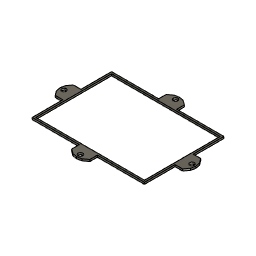
blimp_PCB (Autodesk Fusion 360 archive; units mm, degrees)
design "drzak_kamera"
Autodesk Fusion 360 part; units mm, degrees
(part 1 of 2)
sketch "Sketch1" plane through (0, 0, 0) normal (0, 0, 1) x (1, 0, 0)
  line L0 (29.9, -20.85) -> (-29.9, -20.85)
  line L1 (-29.9, -20.85) -> (-29.9, 20.85)
  line L2 (-29.9, 20.85) -> (29.9, 20.85)
  line L3 (29.9, 20.85) -> (29.9, -20.85)
  line L4 (29.9, -20.85) -> (-29.9, 20.85) construction
  line L5 (-29.9, -20.85) -> (29.9, 20.85) construction
  line L6 (30.9, -21.85) -> (-30.9, -21.85)
  line L7 (-30.9, -21.85) -> (-30.9, 21.85)
  line L8 (-30.9, 21.85) -> (30.9, 21.85)
  line L9 (30.9, 21.85) -> (30.9, -21.85)
  line L10 (30.9, -21.85) -> (-30.9, 21.85) construction
  line L11 (-30.9, -21.85) -> (30.9, 21.85) construction
  dimension "d5" = 41.7
  dimension "d6" = 59.8
  dimension "d8" = 1
  dimension "d9" = 1
  constraint horizontal L0
  constraint perpendicular L0 L1
  constraint parallel L0 L2
  constraint parallel L1 L3
  constraint coincident L4 origin
  constraint coincident L5 origin
  constraint horizontal L6
  constraint perpendicular L6 L7
  constraint parallel L6 L8
  constraint parallel L7 L9
  constraint coincident L10 origin
  constraint coincident L11 origin
  measures "d5" distance of L0 L2
  measures "d6" distance of L1 L3
  measures "d8" distance of L3 L9
  measures "d9" distance of L2 L8
extrude "Extrude1" add sketch "Sketch1" along normal blind 20 makes body 1
extrude "Extrude2" add sketch "Sketch1" against normal blind 1 contours L0 L1 L2 L3 | L6 L7 L8 L9 bodies 1
sketch "Sketch2" plane through (0, 0, -1) normal (0, 0, -1) x (1, 0, 0)
  line L0 (-30.9, -21.85) -> (30.9, -21.85)
  line L1 (30.9, -21.85) -> (30.9, 21.85)
  line L2 (30.9, 21.85) -> (-30.9, 21.85)
  line L3 (-30.9, 21.85) -> (-30.9, -21.85)
  line L4 (29.9, -20.85) -> (29.9, 20.85)
  line L5 (29.9, 20.85) -> (-29.9, 20.85)
  line L6 (-29.9, -20.85) -> (29.9, -20.85)
  line L7 (-29.9, 20.85) -> (-29.9, -20.85)
  circle A0 centre (-14.1, -6.05) radius 10.8
  line L8 (-14.1, -6.05) -> (-14.1, -20.1) construction
  line L9 (-14.1, -6.05) -> (-11.3071, -6.05) construction
  line L10 (-14.1, -6.05) -> (-26.7, -6.05) construction
  point P0 (-14.1, -16.85)
  point P1 (-24.9, -6.05)
  dimension "d16" = 4
  dimension "d18" = 21.6
  dimension "d22" = 5
  constraint coincident A0.centre L8.start
  constraint perpendicular L0 L8
  constraint coincident A0 P0
  constraint coincident L8 P0
  constraint perpendicular L8 L9
  constraint perpendicular L8 L10
  constraint coincident A0 P1
  constraint coincident L10 P1
  measures "d16" distance of L6 P0
  measures "d18" diameter of A0
  measures "d22" distance of L7 P1
extrude "Extrude3" cut sketch "Sketch2" against normal blind 10 contours A0 bodies 1
sketch "Sketch4" plane through (0, 0, 20) normal (0, 0, 1) x (-1, 0, 0)
  line L0 (29.9, -20.85) -> (-29.9, -20.85)
  line L1 (-29.9, -20.85) -> (-29.9, 20.85)
  line L2 (-29.9, 20.85) -> (29.9, 20.85)
  line L3 (29.9, 20.85) -> (29.9, -20.85)
  line L4 (-30.9, -21.85) -> (30.9, -21.85)
  line L5 (30.9, -21.85) -> (30.9, 21.85)
  line L6 (30.9, 21.85) -> (-30.9, 21.85)
  line L7 (-30.9, 21.85) -> (-30.9, -21.85)
  circle A0 centre (0, 21.85) radius 6.5 construction
  line L8 (5, 21.85) -> (5, 29.4381)
  line L9 (0, 21.85) -> (0, 31.6147) construction
  line L10 (-5, 21.85) -> (-5, 29.4381)
  line L11 (0, 0) -> (38, 0) construction
  circle A1 centre (30.9, 0) radius 6.5
  line L12 (30.9, 5) -> (35.0533, 5)
  line L13 (30.9, -5) -> (35.0533, -5)
  circle A2 centre (0, 26.1833) radius 1.25
  line L14 (-30.9, 21.85) -> (30.9, 21.85)
  circle A3 centre (35.2333, 0) radius 1.25
  line L15 (30.9, 21.85) -> (30.9, -21.85)
  line L16 (0, 28.35) -> (2.5, 27.85)
  line L17 (2.5, 27.85) -> (5, 26.0033)
  line L18 (-2.5, 27.85) -> (-5, 26.0033)
  line L19 (0, 28.35) -> (-2.5, 27.85)
  line L20 (37.4, 0) -> (36.9, 2.5)
  line L21 (36.9, 2.5) -> (35.0533, 5)
  line L22 (37.4, 0) -> (36.9, -2.5)
  line L23 (36.9, -2.5) -> (35.0533, -5)
  line L24 (-5, -21.85) -> (-5, -29.4381)
  line L25 (5, -21.85) -> (5, -29.4381)
  line L26 (2.5, -27.85) -> (5, -26.0033)
  line L27 (0, -28.35) -> (2.5, -27.85)
  line L28 (0, -28.35) -> (-2.5, -27.85)
  line L29 (-2.5, -27.85) -> (-5, -26.0033)
  circle A4 centre (0, -26.1833) radius 1.25
  line L30 (0, 0) -> (0, -18) construction
  line L31 (-36.9, -2.5) -> (-35.0533, -5)
  line L32 (-37.4, 0) -> (-36.9, -2.5)
  line L33 (-37.4, 0) -> (-36.9, 2.5)
  line L34 (-36.9, 2.5) -> (-35.0533, 5)
  line L35 (-30.9, 5) -> (-35.0533, 5)
  line L36 (-30.9, -5) -> (-35.0533, -5)
  circle A5 centre (-35.2333, 0) radius 1.25
  dimension "d64" = 13
  dimension "d65" = 5
  dimension "d66" = 5
  dimension "d67" = 13
  dimension "d108" = 4.3333
  dimension "d110" = 4.3333
  dimension "d111" = 2.5
  dimension "d136" = 2.5
  dimension "d137" = 2.5
  dimension "d138" = 2.5
  constraint midpoint L6 A0.centre
  constraint coincident L6 L8.start
  constraint perpendicular L6 L8
  constraint coincident A0.centre L9.start
  constraint perpendicular L6 L9
  constraint symmetric L8.start L9 L10.start
  constraint symmetric L8.end L9 L10.end
  constraint coincident L11.start L30.start
  constraint perpendicular L5 L11
  constraint midpoint L5 A1.centre
  constraint coincident L5 L12.start
  constraint perpendicular L5 L12
  constraint symmetric L11 L12.start L13.start
  constraint symmetric L11 L12.end L13.end
  constraint coincident L9 A2.centre
  constraint coincident L11 A3.centre
  constraint coincident A0 L16.start
  constraint coincident L9 L16.start
  constraint coincident A0 L16.end
  constraint coincident L8 L17.end
  constraint coincident A0 L17.end
  constraint symmetric L9 L16.start L19.start
  constraint symmetric L9 L16.end L18.start
  constraint symmetric L9 L17.end L18.end
  constraint coincident A1 L20.start
  constraint coincident L11 L20.start
  constraint coincident A1 L20.end
  constraint coincident A1 L12.end
  constraint symmetric L11 L20.start L22.start
  constraint symmetric L11 L20.end L22.end
  constraint symmetric L8.start L11 L25.start
  constraint symmetric L8.end L11 L25.end
  constraint symmetric L10.start L11 L24.start
  constraint symmetric L10.end L11 L24.end
  constraint symmetric L11 A2 A4
  constraint symmetric L11 L16.start L27.start
  constraint symmetric L11 L16.end L26.start
  constraint symmetric L11 L17.end L26.end
  constraint symmetric L11 L18.start L28.end
  constraint symmetric L11 L18.end L29.end
  constraint perpendicular L11 L30
  constraint symmetric L12.start L30 L35.start
  constraint symmetric L12.end L30 L34.end
  constraint symmetric L13.start L30 L36.start
  constraint symmetric L13.end L30 L31.end
  constraint symmetric A3 L30 A5
  constraint symmetric L20.start L30 L32.start
  constraint symmetric L20.end L30 L33.end
  constraint symmetric L22.end L30 L31.start
  measures "d64" diameter of A0
  measures "d65" distance of L8 L9
  measures "d66" distance of L11 L12
  measures "d67" diameter of A1
  measures "d108" distance of A2.centre L14
  measures "d110" distance of A3.centre L15
  measures "d111" diameter of A3
  measures "d136" diameter of A2
  measures "d137" horizontal distance of L16.start L16.end
  measures "d138" vertical distance of L20.start L20.end
extrude "Extrude5" add sketch "Sketch4" against normal blind 2 contours L5 L12 L13 L15 L20 L21 L22 L23 | L4 L24 L25 L26 L27 L28 L29 | L6 L8 L10 L14 L16 L17 L18 L19 | L7 L31 L32 L33 L34 L35 L36 bodies 1
sketch "Sketch9" plane through (0, 0, 0) normal (0, 0, 1) x (1, 0, 0)
  circle A0 centre (-14.1, 6.05) radius 10.8
sketch "Sketch11" plane through (0, 0, 0) normal (0, 0, 1) x (-1, 0, 0)
  circle A0 centre (14.1, -6.05) radius 10.8
  line L0 (29.9, -20.85) -> (29.9, 20.85)
  line L1 (29.9, 20.85) -> (-29.9, 20.85)
  line L2 (-29.9, 20.85) -> (-29.9, -20.85)
  line L3 (-29.9, -20.85) -> (29.9, -20.85)
  line L4 (-17.7, -20.85) -> (-17.7, 20.85) construction
  line L5 (-38, -7.65) -> (9, -7.65) construction
  circle A1 centre (-17.7, -7.65) radius 5.5
  dimension "d139" = 12.2
  dimension "d140" = 13.2
  dimension "d141" = 11
  constraint coincident L3 L4.start
  constraint coincident L1 L4.end
  constraint perpendicular L1 L4
  constraint perpendicular L4 L5
  constraint coincident L5 A1.centre
  constraint coincident L4 A1.centre
  measures "d139" distance of L2 L4
  measures "d140" distance of L3 L5
  measures "d141" diameter of A1
extrude "Extrude9" cut sketch "Sketch11" against normal blind 1 contours A1 bodies 1
sketch "Sketch12" plane through (0, 20.85, 0) normal (0, -1, 0) x (1, 0, 0)
  line L0 (-29.9, 0) -> (29.9, 0)
  line L1 (29.9, 0) -> (29.9, 20)
  line L2 (29.9, 20) -> (-29.9, 20)
  line L3 (-29.9, 20) -> (-29.9, 0)
  line L4 (18.2, 24) -> (18.2, -6) construction
  line L5 (6, 12.3) -> (38.4279, 12.3) construction
  circle A0 centre (18.2, 12.3) radius 5.5
  dimension "d144" = 11.7
  dimension "d147" = 12.3
  dimension "d148" = 11
  constraint perpendicular L0 L4
  constraint perpendicular L1 L5
  constraint coincident L5 A0.centre
  constraint coincident L4 A0.centre
  measures "d144" distance of L1 L4
  measures "d147" distance of L0 L5
  measures "d148" diameter of A0
extrude "Extrude10" cut sketch "Sketch12" against normal blind 1 contours A0 bodies 1
sketch "Sketch13" plane through (0, 0, 0) normal (0, 0, 1) x (-1, 0, 0)
  circle A0 centre (-17.7, -7.65) radius 5.5
  circle A1 centre (14.1, -6.05) radius 10.8
  line L0 (29.9, -20.85) -> (29.9, 20.85)
  line L1 (29.9, 20.85) -> (-29.9, 20.85)
  line L2 (-29.9, 20.85) -> (-29.9, -20.85)
  line L3 (-29.9, -20.85) -> (29.9, -20.85)
  circle A2 centre (-17.7, -7.65) radius 5.5
  circle A3 centre (14.1, -6.05) radius 10.8
  circle A4 centre (14.1, -6.05) radius 11.8
  circle A5 centre (-17.7, -7.65) radius 6.5
  line L4 (28.4, -20.85) -> (28.4, 20.85)
  line L5 (25.06, -20.85) -> (25.06, 20.85)
  line L6 (24.31, -20.85) -> (24.31, 20.85) construction
  line L7 (20.22, -20.85) -> (20.22, 20.85)
  line L8 (23.56, -20.85) -> (23.56, 20.85)
  line L9 (19.47, -20.85) -> (19.47, 20.85) construction
  line L10 (18.72, -20.85) -> (18.72, 20.85)
  line L11 (15.38, -20.85) -> (15.38, 20.85)
  line L12 (13.88, -20.85) -> (13.88, 20.85)
  line L13 (10.54, -20.85) -> (10.54, 20.85)
  line L14 (9.79, -20.85) -> (9.79, 20.85) construction
  line L15 (9.04, -20.85) -> (9.04, 20.85)
  line L16 (5.7, -20.85) -> (5.7, 20.85)
  line L17 (4.2, -20.85) -> (4.2, 20.85)
  line L18 (0.86, -20.85) -> (0.86, 20.85)
  line L19 (-0.64, -20.85) -> (-0.64, 20.85)
  line L20 (-3.98, -20.85) -> (-3.98, 20.85)
  line L21 (-5.48, -20.85) -> (-5.48, 20.85)
  line L22 (-8.82, -20.85) -> (-8.82, 20.85)
  line L23 (-9.57, -20.85) -> (-9.57, 20.85) construction
  line L24 (-10.32, -20.85) -> (-10.32, 20.85)
  line L25 (-13.66, -20.85) -> (-13.66, 20.85)
  line L26 (-15.16, -20.85) -> (-15.16, 20.85)
  line L27 (-18.5, -20.85) -> (-18.5, 20.85)
  line L28 (-20, -20.85) -> (-20, 20.85)
  line L29 (-23.34, -20.85) -> (-23.34, 20.85)
  line L30 (-24.84, -20.85) -> (-24.84, 20.85)
  line L31 (-28.18, -20.85) -> (-28.18, 20.85)
  line L32 (29.9, -19.35) -> (-29.9, -19.35)
  line L33 (29.9, -15.825) -> (-29.9, -15.825)
  line L34 (29.9, -15.075) -> (-29.9, -15.075) construction
  line L35 (29.9, -10.8) -> (-29.9, -10.8)
  line L36 (29.9, -14.325) -> (-29.9, -14.325)
  line L37 (29.9, -10.05) -> (-29.9, -10.05) construction
  line L38 (29.9, -9.3) -> (-29.9, -9.3)
  line L39 (29.9, -5.775) -> (-29.9, -5.775)
  line L40 (29.9, -5.025) -> (-29.9, -5.025) construction
  line L41 (29.9, -4.275) -> (-29.9, -4.275)
  line L42 (29.9, -0.75) -> (-29.9, -0.75)
  line L43 (29.9, 0.75) -> (-29.9, 0.75)
  line L44 (29.9, 4.275) -> (-29.9, 4.275)
  line L45 (29.9, 5.025) -> (-29.9, 5.025) construction
  line L46 (29.9, 5.775) -> (-29.9, 5.775)
  line L47 (29.9, 9.3) -> (-29.9, 9.3)
  line L48 (29.9, 10.8) -> (-29.9, 10.8)
  line L49 (29.9, 14.325) -> (-29.9, 14.325)
  line L50 (29.9, 15.825) -> (-29.9, 15.825)
  line L51 (29.9, 19.35) -> (-29.9, 19.35)
  line L52 (29.9, 20.1) -> (-29.9, 20.1) construction
  dimension "d151" = 1
  dimension "d152" = 1
  dimension "d155" = 1.5
  dimension "d156" = 3.34
  dimension "d157" = 0.75
  dimension "d158" = 0.75
  dimension "d159" = 0.75
  dimension "d160" = 0.75
  dimension "d161" = 1.5
  dimension "d162" = 1.5
  dimension "d163" = 3.34
  dimension "d164" = 3.34
  dimension "d165" = 5.06
  dimension "d166" = 3.34
  dimension "d167" = 1.5
  dimension "d168" = 3.525
  dimension "d169" = 0.75
  dimension "d170" = 0.75
  constraint coincident L3 L4.start
  constraint coincident L1 L4.end
  constraint perpendicular L1 L4
  constraint coincident L3 L5.start
  constraint coincident L1 L5.end
  constraint perpendicular L1 L5
  constraint coincident L3 L6.start
  constraint coincident L1 L6.end
  constraint perpendicular L1 L6
  constraint symmetric L4.start L6 L7.start
  constraint symmetric L4.end L6 L7.end
  constraint symmetric L5.start L6 L8.start
  constraint symmetric L5.end L6 L8.end
  constraint coincident L3 L9.start
  constraint coincident L1 L9.end
  constraint perpendicular L1 L9
  constraint symmetric L4.start L9 L13.start
  constraint symmetric L4.end L9 L13.end
  constraint symmetric L5.start L9 L12.start
  constraint symmetric L5.end L9 L12.end
  constraint symmetric L7.start L9 L10.start
  constraint symmetric L7.end L9 L10.end
  constraint symmetric L8.start L9 L11.start
  constraint symmetric L8.end L9 L11.end
  constraint coincident L3 L14.start
  constraint coincident L1 L14.end
  constraint perpendicular L1 L14
  constraint symmetric L4.start L14 L22.start
  constraint symmetric L4.end L14 L22.end
  constraint symmetric L5.start L14 L21.start
  constraint symmetric L5.end L14 L21.end
  constraint symmetric L7.start L14 L19.start
  constraint symmetric L7.end L14 L19.end
  constraint symmetric L8.start L14 L20.start
  constraint symmetric L8.end L14 L20.end
  constraint symmetric L10.start L14 L18.start
  constraint symmetric L10.end L14 L18.end
  constraint symmetric L11.start L14 L17.start
  constraint symmetric L11.end L14 L17.end
  constraint symmetric L12.start L14 L16.start
  constraint symmetric L12.end L14 L16.end
  constraint symmetric L13.start L14 L15.start
  constraint symmetric L13.end L14 L15.end
  constraint coincident L3 L23.start
  constraint coincident L1 L23.end
  constraint perpendicular L1 L23
  constraint symmetric L20.start L23 L26.start
  constraint symmetric L20.end L23 L26.end
  constraint symmetric L21.start L23 L25.start
  constraint symmetric L21.end L23 L25.end
  constraint symmetric L22.start L23 L24.start
  constraint symmetric L22.end L23 L24.end
  constraint coincident L3 L27.start
  constraint coincident L1 L27.end
  constraint perpendicular L1 L27
  constraint coincident L3 L28.start
  constraint coincident L1 L28.end
  constraint perpendicular L1 L28
  constraint coincident L3 L29.start
  constraint coincident L1 L29.end
  constraint perpendicular L1 L29
  constraint coincident L3 L30.start
  constraint coincident L1 L30.end
  constraint perpendicular L1 L30
  constraint coincident L3 L31.start
  constraint coincident L1 L31.end
  constraint perpendicular L1 L31
  constraint coincident L0 L32.start
  constraint coincident L2 L32.end
  constraint perpendicular L2 L32
  constraint coincident L0 L33.start
  constraint coincident L2 L33.end
  constraint perpendicular L2 L33
  constraint coincident L0 L34.start
  constraint coincident L2 L34.end
  constraint perpendicular L2 L34
  constraint symmetric L32.start L34 L35.start
  constraint symmetric L32.end L34 L35.end
  constraint symmetric L33.start L34 L36.start
  constraint symmetric L33.end L34 L36.end
  constraint coincident L0 L37.start
  constraint coincident L2 L37.end
  constraint perpendicular L2 L37
  constraint symmetric L34.start L37 L40.start
  constraint symmetric L34.end L37 L40.end
  constraint symmetric L35.start L37 L38.start
  constraint symmetric L35.end L37 L38.end
  constraint symmetric L36.start L37 L39.start
  constraint symmetric L36.end L37 L39.end
  constraint symmetric L34.start L40 L45.start
  constraint symmetric L34.end L40 L45.end
  constraint symmetric L35.start L40 L43.start
  constraint symmetric L35.end L40 L43.end
  constraint symmetric L36.start L40 L44.start
  constraint symmetric L36.end L40 L44.end
  constraint symmetric L38.start L40 L42.start
  constraint symmetric L38.end L40 L42.end
  constraint symmetric L39.start L40 L41.start
  constraint symmetric L39.end L40 L41.end
  constraint symmetric L37.start L45 L52.start
  constraint symmetric L37.end L45 L52.end
  constraint symmetric L38.start L45 L51.start
  constraint symmetric L38.end L45 L51.end
  constraint symmetric L39.start L45 L50.start
  constraint symmetric L39.end L45 L50.end
  constraint symmetric L41.start L45 L49.start
  constraint symmetric L41.end L45 L49.end
  constraint symmetric L42.start L45 L48.start
  constraint symmetric L42.end L45 L48.end
  constraint symmetric L43.start L45 L47.start
  constraint symmetric L43.end L45 L47.end
  constraint symmetric L44.start L45 L46.start
  constraint symmetric L44.end L45 L46.end
  measures "d155" distance of L0 L4
  measures "d156" distance of L4 L5
  measures "d157" distance of L5 L6
  measures "d158" distance of L7 L9
  measures "d159" distance of L13 L14
  measures "d160" distance of L22 L23
  measures "d161" distance of L27 L28
  measures "d162" distance of L29 L30
  measures "d163" distance of L26 L27
  measures "d164" distance of L28 L29
  measures "d165" distance of L2 L30
  measures "d166" distance of L30 L31
  measures "d167" distance of L3 L32
  measures "d168" distance of L32 L33
  measures "d169" distance of L33 L34
  measures "d170" distance of L35 L37
extrude "Extrude11" cut sketch "Sketch13" against normal blind 1 contours A5 L24 L38 L39 | A5 L24 L25 L41 L42 | A5 L24 L25 L35 L36 | L21 L22 L38 L39 | A5 L26 L27 L42 | L21 L22 L41 L42 | A5 L26 L27 L36 | L21 L22 L35 L36 | L24 L25 L43 L44 | L19 L20 L38 L39 | L24 L25 L32 L33 | A5 L28 L29 L41 L42 | L26 L27 L43 L44 | L21 L22 L43 L44 | L19 L20 L41 L42 | A5 L28 L29 L36 | L26 L27 L32 L33 | L21 L22 L32 L33 | L19 L20 L35 L36 | L24 L25 L46 L47 | A4 L18 L38 L39 | L28 L29 L43 L44 | L26 L27 L46 L47 | L21 L22 L46 L47 | L19 L20 L43 L44 | A4 L18 L41 L42 | L30 L31 L38 L39 | L28 L29 L32 L33 | L19 L20 L32 L33 | A4 L17 L18 L35 L36 | L30 L31 L41 L42 | L24 L25 L48 L49 | L30 L31 L35 L36 | L28 L29 L46 L47 | L30 L31 L43 L44 | L26 L27 L48 L49 | L21 L22 L48 L49 | L19 L20 L46 L47 | L17 L18 L43 L44 | L30 L31 L32 L33 | L17 L18 L32 L33 | L24 L25 L50 L51 | L28 L29 L48 L49 | L30 L31 L46 L47 | L26 L27 L50 L51 | L21 L22 L50 L51 | L19 L20 L48 L49 | L17 L18 L46 L47 | A4 L15 L16 L32 L33 | A4 L16 L44 | L28 L29 L50 L51 | L30 L31 L48 L49 | L19 L20 L50 L51 | L17 L18 L48 L49 | L15 L16 L46 L47 | A4 L12 L13 L32 | L30 L31 L50 L51 | L17 L18 L50 L51 | L15 L16 L48 L49 | L12 L13 L46 L47 | A4 L10 L11 L32 | L15 L16 L50 L51 | L12 L13 L48 L49 | L10 L11 L46 L47 | A4 L7 L8 L32 L33 | L12 L13 L50 L51 | L10 L11 L48 L49 | L7 L8 L46 L47 | A4 L7 L8 L44 | A4 L4 L38 L39 | L4 L5 L32 L33 | A4 L8 L36 | L10 L11 L50 L51 | L7 L8 L48 L49 | L4 L5 L46 L47 | A4 L4 L5 L41 L42 | L4 L5 L35 L36 | L4 L5 L43 L44 | L7 L8 L50 L51 | L4 L5 L48 L49 | L4 L5 L50 L51 bodies 1
sketch "Sketch14" plane through (0, 20.85, 0) normal (0, -1, 0) x (1, 0, 0)
  circle A0 centre (18.2, 12.3) radius 5.5
  line L0 (-29.9, 0) -> (29.9, 0)
  line L1 (29.9, 0) -> (29.9, 20)
  line L2 (29.9, 20) -> (-29.9, 20)
  line L3 (-29.9, 20) -> (-29.9, 0)
  line L4 (5, 18) -> (5, 20)
  line L5 (-5, 18) -> (5, 18)
  line L6 (-5, 20) -> (-5, 18)
  line L7 (-6, 20) -> (-6, 17)
  line L8 (-6, 17) -> (6, 17)
  line L9 (6, 17) -> (6, 20)
  circle A1 centre (18.2, 12.3) radius 6.5
  line L10 (-29.9, 18.5) -> (29.9, 18.5)
  line L11 (-29.9, 15.375) -> (29.9, 15.375)
  line L12 (-29.9, 14.625) -> (29.9, 14.625) construction
  line L13 (-29.9, 13.875) -> (29.9, 13.875)
  line L14 (-29.9, 10.75) -> (29.9, 10.75)
  line L15 (-29.9, 10) -> (29.9, 10) construction
  line L16 (-29.9, 9.25) -> (29.9, 9.25)
  line L17 (-29.9, 6.125) -> (29.9, 6.125)
  line L18 (-29.9, 5.375) -> (29.9, 5.375) construction
  line L19 (-29.9, 4.625) -> (29.9, 4.625)
  line L20 (-29.9, 1.5) -> (29.9, 1.5)
  line L21 (-28.4, 20) -> (-28.4, 0)
  line L22 (-25.06, 20) -> (-25.06, 0)
  line L23 (-24.31, 20) -> (-24.31, 0) construction
  line L24 (-20.22, 20) -> (-20.22, 0)
  line L25 (-23.56, 20) -> (-23.56, 0)
  line L26 (-19.47, 20) -> (-19.47, 0) construction
  line L27 (-18.72, 20) -> (-18.72, 0)
  line L28 (-15.38, 20) -> (-15.38, 0)
  line L29 (-14.63, 20) -> (-14.63, 0) construction
  line L30 (-13.88, 20) -> (-13.88, 0)
  line L31 (-10.54, 20) -> (-10.54, 0)
  line L32 (-9.04, 20) -> (-9.04, 0)
  line L33 (-5.7, 20) -> (-5.7, 0)
  line L34 (-4.95, 20) -> (-4.95, 0) construction
  line L35 (-4.2, 20) -> (-4.2, 0)
  line L36 (-0.86, 20) -> (-0.86, 0)
  line L37 (0.64, 20) -> (0.64, 0)
  line L38 (3.98, 20) -> (3.98, 0)
  line L39 (5.48, 20) -> (5.48, 0)
  line L40 (8.82, 20) -> (8.82, 0)
  line L41 (10.32, 20) -> (10.32, 0)
  line L42 (13.66, 20) -> (13.66, 0)
  line L43 (14.41, 20) -> (14.41, 0) construction
  line L44 (15.16, 20) -> (15.16, 0)
  line L45 (18.5, 20) -> (18.5, 0)
  line L46 (20, 20) -> (20, 0)
  line L47 (23.34, 20) -> (23.34, 0)
  line L48 (24.84, 20) -> (24.84, 0)
  line L49 (28.18, 20) -> (28.18, 0)
  dimension "d175" = 1
  dimension "d176" = 1
  dimension "d177" = 1.5
  dimension "d178" = 3.125
  dimension "d180" = 0.75
  dimension "d181" = 0.75
  dimension "d182" = 1.5
  dimension "d183" = 0.75
  dimension "d184" = 3.34
  dimension "d185" = 1.5
  dimension "d186" = 0.75
  dimension "d187" = 1.72
  constraint coincident L3 L10.start
  constraint coincident L1 L10.end
  constraint perpendicular L1 L10
  constraint coincident L3 L11.start
  constraint coincident L1 L11.end
  constraint perpendicular L1 L11
  constraint coincident L3 L12.start
  constraint coincident L1 L12.end
  constraint perpendicular L1 L12
  constraint symmetric L10.start L12 L14.start
  constraint symmetric L10.end L12 L14.end
  constraint symmetric L11.start L12 L13.start
  constraint symmetric L11.end L12 L13.end
  constraint coincident L3 L15.start
  constraint coincident L1 L15.end
  constraint perpendicular L1 L15
  constraint symmetric L12.start L15 L18.start
  constraint symmetric L12.end L15 L18.end
  constraint symmetric L13.start L15 L17.start
  constraint symmetric L13.end L15 L17.end
  constraint symmetric L14.start L15 L16.start
  constraint symmetric L14.end L15 L16.end
  constraint symmetric L16.start L18 L20.start
  constraint symmetric L16.end L18 L20.end
  constraint symmetric L17.start L18 L19.start
  constraint symmetric L17.end L18 L19.end
  constraint coincident L2 L21.start
  constraint coincident L0 L21.end
  constraint perpendicular L0 L21
  constraint coincident L2 L22.start
  constraint coincident L0 L22.end
  constraint perpendicular L0 L22
  constraint coincident L2 L23.start
  constraint coincident L0 L23.end
  constraint perpendicular L0 L23
  constraint symmetric L21.start L23 L24.start
  constraint symmetric L21.end L23 L24.end
  constraint symmetric L22.start L23 L25.start
  constraint symmetric L22.end L23 L25.end
  constraint coincident L2 L26.start
  constraint coincident L0 L26.end
  constraint perpendicular L0 L26
  constraint symmetric L23.start L26 L29.start
  constraint symmetric L23.end L26 L29.end
  constraint symmetric L24.start L26 L27.start
  constraint symmetric L24.end L26 L27.end
  constraint symmetric L25.start L26 L28.start
  constraint symmetric L25.end L26 L28.end
  constraint symmetric L23.start L29 L34.start
  constraint symmetric L23.end L29 L34.end
  constraint symmetric L24.start L29 L32.start
  constraint symmetric L24.end L29 L32.end
  constraint symmetric L25.start L29 L33.start
  constraint symmetric L25.end L29 L33.end
  constraint symmetric L27.start L29 L31.start
  constraint symmetric L27.end L29 L31.end
  constraint symmetric L28.start L29 L30.start
  constraint symmetric L28.end L29 L30.end
  constraint symmetric L23.start L34 L43.start
  constraint symmetric L23.end L34 L43.end
  constraint symmetric L24.start L34 L41.start
  constraint symmetric L24.end L34 L41.end
  constraint symmetric L25.start L34 L42.start
  constraint symmetric L25.end L34 L42.end
  constraint symmetric L27.start L34 L40.start
  constraint symmetric L27.end L34 L40.end
  constraint symmetric L28.start L34 L39.start
  constraint symmetric L28.end L34 L39.end
  constraint symmetric L30.start L34 L38.start
  constraint symmetric L30.end L34 L38.end
  constraint symmetric L31.start L34 L37.start
  constraint symmetric L31.end L34 L37.end
  constraint symmetric L32.start L34 L36.start
  constraint symmetric L32.end L34 L36.end
  constraint symmetric L33.start L34 L35.start
  constraint symmetric L33.end L34 L35.end
  constraint symmetric L37.start L43 L49.start
  constraint symmetric L37.end L43 L49.end
  constraint symmetric L38.start L43 L48.start
  constraint symmetric L38.end L43 L48.end
  constraint symmetric L39.start L43 L47.start
  constraint symmetric L39.end L43 L47.end
  constraint symmetric L40.start L43 L46.start
  constraint symmetric L40.end L43 L46.end
  constraint symmetric L41.start L43 L45.start
  constraint symmetric L41.end L43 L45.end
  constraint symmetric L42.start L43 L44.start
  constraint symmetric L42.end L43 L44.end
  measures "d177" distance of L2 L10
  measures "d178" distance of L10 L11
  measures "d180" distance of L11 L12
  measures "d181" distance of L14 L15
  measures "d182" distance of L0 L20
  measures "d183" distance of L22 L23
  measures "d184" distance of L21 L22
  measures "d185" distance of L3 L21
  measures "d186" distance of L24 L26
  measures "d187" distance of L1 L49
extrude "Extrude12" cut sketch "Sketch14" against normal blind 1 contours L13 L14 L48 L49 | A1 L10 L47 | L10 L11 L48 L49 | A1 L17 L47 | L16 L17 L48 L49 | L19 L20 L46 L47 | L19 L20 L48 L49 | A1 L10 L44 | A1 L10 L11 L41 L42 | A1 L13 L14 L41 | A1 L16 L17 L41 L42 | L19 L20 L44 L45 | L13 L14 L39 L40 | L19 L20 L41 L42 | L8 L9 L10 L11 L39 L40 | L16 L17 L39 L40 | L13 L14 L37 L38 | L19 L20 L39 L40 | L8 L11 L37 L38 | L16 L17 L37 L38 | L13 L14 L35 L36 | L19 L20 L37 L38 | L8 L11 L35 L36 | L16 L17 L35 L36 | L13 L14 L32 L33 | L19 L20 L35 L36 | L7 L8 L10 L11 L32 L33 | L16 L17 L32 L33 | L13 L14 L30 L31 | L19 L20 L32 L33 | L10 L11 L30 L31 | L16 L17 L30 L31 | L13 L14 L27 L28 | L19 L20 L30 L31 | L10 L11 L27 L28 | L16 L17 L27 L28 | L13 L14 L24 L25 | L19 L20 L27 L28 | L10 L11 L24 L25 | L16 L17 L24 L25 | L13 L14 L21 L22 | L19 L20 L24 L25 | L10 L11 L21 L22 | L16 L17 L21 L22 | L19 L20 L21 L22 bodies 1
sketch "Sketch15" plane through (0, -20.85, 0) normal (0, 1, 0) x (-1, 0, 0)
  line L0 (-29.9, 0) -> (29.9, 0)
  line L1 (29.9, 0) -> (29.9, 20)
  line L2 (29.9, 20) -> (-29.9, 20)
  line L3 (-29.9, 20) -> (-29.9, 0)
  line L4 (-29.9, 18.5) -> (-28, 18.5)
  line L5 (-28, 18.5) -> (29.9, 18.5)
  line L6 (-29.9, 15.375) -> (29.9, 15.375)
  line L7 (-29.9, 13.875) -> (29.9, 13.875)
  line L8 (-29.9, 10.75) -> (29.9, 10.75)
  line L9 (-29.9, 14.625) -> (29.9, 14.625) construction
  line L10 (-29.9, 10) -> (29.9, 10) construction
  line L11 (-29.9, 9.25) -> (29.9, 9.25)
  line L12 (-29.9, 6.125) -> (29.9, 6.125)
  line L13 (-29.9, 5.375) -> (29.9, 5.375) construction
  line L14 (-29.9, 4.625) -> (29.9, 4.625)
  line L15 (-29.9, 1.5) -> (29.9, 1.5)
  line L16 (-28.4, 20) -> (-28.4, 0)
  line L17 (-25.06, 20) -> (-25.06, 0)
  line L18 (-23.56, 20) -> (-23.56, 0)
  line L19 (-20.22, 20) -> (-20.22, 0)
  line L20 (-19.47, 0) -> (-19.47, 20) construction
  line L21 (-29.15, 0) -> (-29.15, 20) construction
  line L22 (-18.72, 20) -> (-18.72, 0)
  line L23 (-15.38, 20) -> (-15.38, 0)
  line L24 (-13.88, 20) -> (-13.88, 0)
  line L25 (-10.54, 20) -> (-10.54, 0)
  line L26 (-9.79, 0) -> (-9.79, 20) construction
  line L27 (-9.04, 20) -> (-9.04, 0)
  line L28 (-5.7, 20) -> (-5.7, 0)
  line L29 (-4.2, 20) -> (-4.2, 0)
  line L30 (-0.86, 20) -> (-0.86, 0)
  line L31 (0.64, 20) -> (0.64, 0)
  line L32 (3.98, 20) -> (3.98, 0)
  line L33 (5.48, 20) -> (5.48, 0)
  line L34 (8.82, 20) -> (8.82, 0)
  line L35 (9.57, 0) -> (9.57, 20) construction
  line L36 (10.32, 20) -> (10.32, 0)
  line L37 (13.66, 20) -> (13.66, 0)
  line L38 (15.16, 20) -> (15.16, 0)
  line L39 (18.5, 20) -> (18.5, 0)
  line L40 (20, 20) -> (20, 0)
  line L41 (23.34, 20) -> (23.34, 0)
  line L42 (24.84, 20) -> (24.84, 0)
  line L43 (28.18, 20) -> (28.18, 0)
  line L44 (-5, 18) -> (5, 18)
  line L45 (5, 18) -> (5, 20)
  line L46 (-5, 20) -> (-5, 18)
  line L47 (-6, 20) -> (-6, 17)
  line L48 (-6, 17) -> (6, 17)
  line L49 (6, 17) -> (6, 20)
  dimension "d190" = 1.5
  dimension "d191" = 3.125
  dimension "d192" = 1.5
  dimension "d193" = 3.125
  dimension "d194" = 0.75
  dimension "d195" = 0.75
  dimension "d196" = 1.5
  dimension "d197" = 3.34
  dimension "d198" = 1.5
  dimension "d199" = 3.34
  dimension "d200" = 0.75
  dimension "d201" = 0.75
  dimension "d204" = 1
  constraint coincident L3 L4.start
  constraint perpendicular L3 L4
  constraint coincident L1 L5.end
  constraint perpendicular L1 L5
  constraint coincident L3 L6.start
  constraint coincident L1 L6.end
  constraint perpendicular L3 L6
  constraint coincident L3 L7.start
  constraint perpendicular L3 L7
  constraint coincident L3 L8.start
  constraint coincident L1 L8.end
  constraint perpendicular L1 L8
  constraint coincident L3 L9.start
  constraint coincident L1 L9.end
  constraint perpendicular L1 L9
  constraint coincident L3 L10.start
  constraint coincident L1 L10.end
  constraint perpendicular L1 L10
  constraint symmetric L7.start L10 L12.start
  constraint symmetric L7.end L10 L12.end
  constraint symmetric L8.start L10 L11.start
  constraint symmetric L8.end L10 L11.end
  constraint symmetric L9.start L10 L13.start
  constraint symmetric L9.end L10 L13.end
  constraint symmetric L11.start L13 L15.start
  constraint symmetric L11.end L13 L15.end
  constraint symmetric L12.start L13 L14.start
  constraint symmetric L12.end L13 L14.end
  constraint coincident L2 L16.start
  constraint coincident L0 L16.end
  constraint perpendicular L0 L16
  constraint coincident L2 L17.start
  constraint coincident L0 L17.end
  constraint perpendicular L0 L17
  constraint coincident L2 L18.start
  constraint coincident L0 L18.end
  constraint perpendicular L0 L18
  constraint coincident L2 L19.start
  constraint coincident L0 L19.end
  constraint perpendicular L0 L19
  constraint coincident L0 L20.start
  constraint coincident L2 L20.end
  constraint perpendicular L2 L20
  constraint coincident L0 L21.start
  constraint coincident L2 L21.end
  constraint perpendicular L2 L21
  constraint symmetric L16.start L20 L25.start
  constraint symmetric L16.end L20 L25.end
  constraint symmetric L17.start L20 L24.start
  constraint symmetric L17.end L20 L24.end
  constraint symmetric L18.start L20 L23.start
  constraint symmetric L18.end L20 L23.end
  constraint symmetric L19.start L20 L22.start
  constraint symmetric L19.end L20 L22.end
  constraint symmetric L20 L21.start L26.start
  constraint symmetric L20 L21.end L26.end
  constraint symmetric L16.start L26 L34.start
  constraint symmetric L16.end L26 L34.end
  constraint symmetric L17.start L26 L33.start
  constraint symmetric L17.end L26 L33.end
  constraint symmetric L18.start L26 L32.start
  constraint symmetric L18.end L26 L32.end
  constraint symmetric L19.start L26 L31.start
  constraint symmetric L19.end L26 L31.end
  constraint symmetric L21.start L26 L35.start
  constraint symmetric L21.end L26 L35.end
  constraint symmetric L22.start L26 L30.start
  constraint symmetric L22.end L26 L30.end
  constraint symmetric L23.start L26 L29.start
  constraint symmetric L23.end L26 L29.end
  constraint symmetric L24.start L26 L28.start
  constraint symmetric L24.end L26 L28.end
  constraint symmetric L25.start L26 L27.start
  constraint symmetric L25.end L26 L27.end
  constraint symmetric L27.start L35 L43.start
  constraint symmetric L27.end L35 L43.end
  constraint symmetric L28.start L35 L42.start
  constraint symmetric L28.end L35 L42.end
  constraint symmetric L29.start L35 L41.start
  constraint symmetric L29.end L35 L41.end
  constraint symmetric L30.start L35 L40.start
  constraint symmetric L30.end L35 L40.end
  constraint symmetric L31.start L35 L39.start
  constraint symmetric L31.end L35 L39.end
  constraint symmetric L32.start L35 L38.start
  constraint symmetric L32.end L35 L38.end
  constraint symmetric L33.start L35 L37.start
  constraint symmetric L33.end L35 L37.end
  constraint symmetric L34.start L35 L36.start
  constraint symmetric L34.end L35 L36.end
  measures "d190" distance of L2 L5
  measures "d191" distance of L5 L6
  measures "d192" distance of L6 L7
  measures "d193" distance of L7 L8
  measures "d194" distance of L6 L9
  measures "d195" distance of L8 L10
  measures "d196" distance of L3 L16
  measures "d197" distance of L16 L17
  measures "d198" distance of L17 L18
  measures "d199" distance of L18 L19
  measures "d200" distance of L16 L21
  measures "d201" distance of L19 L20
extrude "Extrude13" cut sketch "Sketch15" against normal blind 1 contours L14 L15 L16 L17 | L14 L15 L18 L19 | L11 L12 L16 L17 | L14 L15 L22 L23 | L11 L12 L18 L19 | L7 L8 L16 L17 | L14 L15 L24 L25 | L11 L12 L22 L23 | L7 L8 L18 L19 | L4 L5 L6 L16 L17 | L14 L15 L27 L28 | L11 L12 L24 L25 | L7 L8 L22 L23 | L5 L6 L18 L19 | L14 L15 L29 L30 | L11 L12 L27 L28 | L7 L8 L24 L25 | L5 L6 L22 L23 | L14 L15 L31 L32 | L11 L12 L29 L30 | L7 L8 L27 L28 | L5 L6 L24 L25 | L14 L15 L33 L34 | L11 L12 L31 L32 | L7 L8 L29 L30 | L5 L6 L27 L28 L47 L48 | L14 L15 L36 L37 | L11 L12 L33 L34 | L7 L8 L31 L32 | L6 L29 L30 L48 | L14 L15 L38 L39 | L11 L12 L36 L37 | L7 L8 L33 L34 | L6 L31 L32 L48 | L14 L15 L40 L41 | L11 L12 L38 L39 | L7 L8 L36 L37 | L5 L6 L33 L34 L48 L49 | L14 L15 L42 L43 | L11 L12 L40 L41 | L7 L8 L38 L39 | L5 L6 L36 L37 | L11 L12 L42 L43 | L5 L6 L38 L39 | L7 L8 L42 L43 | L5 L6 L40 L41 | L5 L6 L42 L43 bodies 1
sketch "Sketch16" plane through (29.9, 0, 0) normal (-1, 0, 0) x (0, -1, 0)
  line L0 (-20.85, 0) -> (20.85, 0)
  line L1 (20.85, 0) -> (20.85, 20)
  line L2 (20.85, 20) -> (-20.85, 20)
  line L3 (-20.85, 20) -> (-20.85, 0)
  line L4 (5, 18) -> (5, 20)
  line L5 (-5, 18) -> (5, 18)
  line L6 (-5, 20) -> (-5, 18)
  line L7 (-6, 20) -> (-6, 17)
  line L8 (-6, 17) -> (6, 17)
  line L9 (6, 17) -> (6, 20)
  line L10 (-20.85, 18.5) -> (20.85, 18.5)
  line L11 (-20.85, 15.375) -> (20.85, 15.375)
  line L12 (20.85, 14.625) -> (20, 14.625) construction
  line L13 (20, 14.625) -> (-20.85, 14.625) construction
  line L14 (-20.85, 10.75) -> (20.85, 10.75)
  line L15 (-20.85, 13.875) -> (20.85, 13.875)
  line L16 (20.85, 10) -> (-20.85, 10) construction
  line L17 (-20.85, 9.25) -> (20.85, 9.25)
  line L18 (-20.85, 6.125) -> (20.85, 6.125)
  line L19 (20, 5.375) -> (-20.85, 5.375) construction
  line L20 (-20.85, 4.625) -> (20.85, 4.625)
  line L21 (-20.85, 1.5) -> (20.85, 1.5)
  line L22 (-19.35, 20) -> (-19.35, 0)
  line L23 (-15.825, 20) -> (-15.825, 0)
  line L24 (-15.075, 20) -> (-15.075, 0) construction
  line L25 (-14.325, 20) -> (-14.325, 0)
  line L26 (-10.8, 20) -> (-10.8, 0)
  line L27 (-10.05, 20) -> (-10.05, 0) construction
  line L28 (-9.3, 20) -> (-9.3, 0)
  line L29 (-5.775, 20) -> (-5.775, 0)
  line L30 (-5.025, 20) -> (-5.025, 0) construction
  line L31 (-4.275, 20) -> (-4.275, 0)
  line L32 (-0.75, 20) -> (-0.75, 0)
  line L33 (0.75, 20) -> (0.75, 0)
  line L34 (4.275, 20) -> (4.275, 0)
  line L35 (5.025, 20) -> (5.025, 0) construction
  line L36 (5.775, 20) -> (5.775, 0)
  line L37 (9.3, 20) -> (9.3, 0)
  line L38 (10.8, 20) -> (10.8, 0)
  line L39 (14.325, 20) -> (14.325, 0)
  line L40 (15.825, 20) -> (15.825, 0)
  line L41 (19.35, 20) -> (19.35, 0)
  dimension "d205" = 1
  dimension "d206" = 1.5
  dimension "d207" = 3.125
  dimension "d208" = 0.75
  dimension "d209" = 0.75
  dimension "d210" = 1.5
  dimension "d211" = 3.525
  dimension "d212" = 0.75
  dimension "d213" = 0.75
  constraint coincident L3 L10.start
  constraint coincident L1 L10.end
  constraint perpendicular L1 L10
  constraint coincident L3 L11.start
  constraint coincident L1 L11.end
  constraint perpendicular L1 L11
  constraint coincident L1 L12.start
  constraint perpendicular L1 L12
  constraint coincident L3 L13.end
  constraint perpendicular L3 L13
  constraint symmetric L10.start L13 L14.start
  constraint symmetric L10.end L13 L14.end
  constraint symmetric L11.start L13 L15.start
  constraint symmetric L11.end L13 L15.end
  constraint coincident L1 L16.start
  constraint coincident L3 L16.end
  constraint perpendicular L3 L16
  constraint symmetric L12.end L16 L19.start
  constraint symmetric L13.end L16 L19.end
  constraint symmetric L14.start L16 L17.start
  constraint symmetric L14.end L16 L17.end
  constraint symmetric L15.start L16 L18.start
  constraint symmetric L15.end L16 L18.end
  constraint symmetric L17.start L19 L21.start
  constraint symmetric L17.end L19 L21.end
  constraint symmetric L18.start L19 L20.start
  constraint symmetric L18.end L19 L20.end
  constraint coincident L2 L22.start
  constraint coincident L0 L22.end
  constraint perpendicular L0 L22
  constraint coincident L2 L23.start
  constraint coincident L0 L23.end
  constraint perpendicular L0 L23
  constraint coincident L2 L24.start
  constraint coincident L0 L24.end
  constraint perpendicular L0 L24
  constraint symmetric L22.start L24 L26.start
  constraint symmetric L22.end L24 L26.end
  constraint symmetric L23.start L24 L25.start
  constraint symmetric L23.end L24 L25.end
  constraint coincident L0 L27.end
  constraint perpendicular L0 L27
  constraint symmetric L24.start L27 L30.start
  constraint symmetric L24.end L27 L30.end
  constraint symmetric L25.start L27 L29.start
  constraint symmetric L25.end L27 L29.end
  constraint symmetric L26.start L27 L28.start
  constraint symmetric L26.end L27 L28.end
  constraint symmetric L24.start L30 L35.start
  constraint symmetric L24.end L30 L35.end
  constraint symmetric L25.start L30 L34.start
  constraint symmetric L25.end L30 L34.end
  constraint symmetric L26.start L30 L33.start
  constraint symmetric L26.end L30 L33.end
  constraint symmetric L28.start L30 L32.start
  constraint symmetric L28.end L30 L32.end
  constraint symmetric L29.start L30 L31.start
  constraint symmetric L29.end L30 L31.end
  constraint symmetric L28.start L35 L41.start
  constraint symmetric L28.end L35 L41.end
  constraint symmetric L29.start L35 L40.start
  constraint symmetric L29.end L35 L40.end
  constraint symmetric L31.start L35 L39.start
  constraint symmetric L31.end L35 L39.end
  constraint symmetric L32.start L35 L38.start
  constraint symmetric L32.end L35 L38.end
  constraint symmetric L33.start L35 L37.start
  constraint symmetric L33.end L35 L37.end
  constraint symmetric L34.start L35 L36.start
  constraint symmetric L34.end L35 L36.end
  measures "d206" distance of L2 L10
  measures "d207" distance of L10 L11
  measures "d208" distance of L11 L13
  measures "d209" distance of L14 L16
  measures "d210" distance of L3 L22
  measures "d211" distance of L22 L23
  measures "d212" distance of L23 L24
  measures "d213" distance of L26 L27
extrude "Extrude14" cut sketch "Sketch16" along normal blind -1 and the other way blind -60.8 contours L20 L21 L22 L23 | L20 L21 L25 L26 | L17 L18 L22 L23 | L20 L21 L28 L29 | L17 L18 L25 L26 | L14 L15 L22 L23 | L20 L21 L31 L32 | L17 L18 L28 L29 | L14 L15 L25 L26 | L10 L11 L22 L23 | L20 L21 L33 L34 | L17 L18 L31 L32 | L14 L15 L28 L29 | L10 L11 L25 L26 | L20 L21 L36 L37 | L17 L18 L33 L34 | L14 L15 L31 L32 | L7 L8 L10 L11 L28 L29 | L20 L21 L38 L39 | L17 L18 L36 L37 | L14 L15 L33 L34 | L8 L11 L31 L32 | L20 L21 L40 L41 | L17 L18 L38 L39 | L14 L15 L36 L37 | L8 L11 L33 L34 | L17 L18 L40 L41 | L14 L15 L38 L39 | L8 L9 L10 L11 L36 L37 | L14 L15 L40 L41 | L10 L11 L38 L39 | L10 L11 L40 L41 bodies 1
sketch "Sketch17" plane through (0, 0, 20) normal (0, 0, 1) x (-1, 0, 0)
  circle A0 centre (-35.2333, 0) radius 1.25
  circle A1 centre (0, -26.1833) radius 1.25
  circle A2 centre (0, 26.1833) radius 1.25
  circle A3 centre (35.2333, 0) radius 1.25
  line L0 (29.9, -20.85) -> (-29.9, -20.85)
  line L1 (-29.9, -20.85) -> (-29.9, 20.85)
  line L2 (-29.9, 20.85) -> (29.9, 20.85)
  line L3 (29.9, 20.85) -> (29.9, -20.85)
  line L4 (-30.9, -21.85) -> (-5, -21.85)
  line L5 (-5, -21.85) -> (-5, -26.0033)
  line L6 (-5, -26.0033) -> (-2.5, -27.85)
  line L7 (-2.5, -27.85) -> (0, -28.35)
  line L8 (0, -28.35) -> (2.5, -27.85)
  line L9 (2.5, -27.85) -> (5, -26.0033)
  line L10 (5, -26.0033) -> (5, -21.85)
  line L11 (5, -21.85) -> (30.9, -21.85)
  line L12 (30.9, -21.85) -> (30.9, -5)
  line L13 (30.9, -5) -> (35.0533, -5)
  line L14 (35.0533, -5) -> (36.9, -2.5)
  line L15 (36.9, -2.5) -> (37.4, 0)
  line L16 (37.4, 0) -> (36.9, 2.5)
  line L17 (36.9, 2.5) -> (35.0533, 5)
  line L18 (35.0533, 5) -> (30.9, 5)
  line L19 (30.9, 5) -> (30.9, 21.85)
  line L20 (30.9, 21.85) -> (5, 21.85)
  line L21 (5, 21.85) -> (5, 26.0033)
  line L22 (5, 26.0033) -> (2.5, 27.85)
  line L23 (2.5, 27.85) -> (0, 28.35)
  line L24 (0, 28.35) -> (-2.5, 27.85)
  line L25 (-2.5, 27.85) -> (-5, 26.0033)
  line L26 (-5, 26.0033) -> (-5, 21.85)
  line L27 (-5, 21.85) -> (-30.9, 21.85)
  line L28 (-30.9, 21.85) -> (-30.9, 5)
  line L29 (-30.9, 5) -> (-35.0533, 5)
  line L30 (-35.0533, 5) -> (-36.9, 2.5)
  line L31 (-36.9, 2.5) -> (-37.4, 0)
  line L32 (-37.4, 0) -> (-36.9, -2.5)
  line L33 (-36.9, -2.5) -> (-35.0533, -5)
  line L34 (-35.0533, -5) -> (-30.9, -5)
  line L35 (-30.9, -5) -> (-30.9, -21.85)
extrude "Extrude1'" add sketch "Sketch17" along normal blind 1 separate body makes body 2 in component "Component"
component "Component" placed x (1, 0, 0) y (0, 1, 0) z (0, 0, 1) at (0, 0, 0)
equation "kamera_vyska = 41.7 mm"
equation "kamera_sirka = 59.8 mm"
equation "odstup_cocka_zvrchu = 4 mm"
equation "odstup_cocka_zboku = 5 mm"
equation "d5 = kamera_vyska"
equation "d6 = kamera_sirka"
equation "okraj = 1 mm"
equation "d8 = okraj"
equation "d9 = okraj"
equation "hloubka_drzak = 20 mm"
equation "d11 = hloubka_drzak"
equation "d13 = -okraj"
equation "d18 = velikost_cocky"
equation "velikost_cocky = 21.6 mm"
equation "d22 = odstup_cocka_zboku"
equation "pricka = 1.5 mm"
equation "sirka_uchyceni = 5 mm"
equation "prumer_uchyceni = 13 mm"
equation "d64 = prumer_uchyceni"
equation "d65 = sirka_uchyceni"
equation "d66 = sirka_uchyceni"
equation "d67 = prumer_uchyceni"
equation "uchyceni_hloubka = 2 mm"
equation "d108 = d64 / 3"
equation "uchycujici_dira = uchycujici_diraa"
equation "d110 = d67 / 3"
equation "d111 = uchycujici_dira"
equation "uchycujici_diraa = 2.5 mm"
equation "d136 = uchycujici_diraa"
equation "d137 = sirka_uchyceni / 2"
equation "d138 = sirka_uchyceni / 2"
equation "d142 = -okraj"
equation "d149 = -okraj"
equation "mriz_y = 3.525 mm"
equation "mriz_x = 3.34 mm"
equation "d155 = pricka"
equation "d156 = mriz_x"
equation "d157 = pricka / 2"
equation "d158 = pricka / 2"
equation "d159 = pricka / 2"
equation "d160 = pricka / 2"
equation "d161 = pricka"
equation "d162 = pricka"
equation "d163 = mriz_x"
equation "d164 = mriz_x"
equation "d166 = mriz_x"
equation "d167 = pricka"
equation "d168 = mriz_y"
equation "d169 = pricka / 2"
equation "d170 = pricka / 2"
equation "d172 = -okraj"
equation "d177 = pricka"
equation "d178 = mriz_z"
equation "mriz_z = 3.125 mm"
equation "d180 = pricka / 2"
equation "d181 = pricka / 2"
equation "d183 = pricka / 2"
equation "d184 = mriz_x"
equation "d185 = pricka"
equation "d186 = pricka / 2"
equation "d188 = -okraj"
equation "d190 = pricka"
equation "d191 = mriz_z"
equation "d192 = pricka"
equation "d193 = mriz_z"
equation "d194 = pricka / 2"
equation "d195 = pricka / 2"
equation "d196 = pricka"
equation "d197 = mriz_x"
equation "d198 = pricka"
equation "d199 = mriz_x"
equation "d200 = pricka / 2"
equation "d201 = pricka / 2"
equation "d202 = -okraj"
equation "d206 = pricka"
equation "d207 = mriz_z"
equation "d208 = pricka / 2"
equation "d209 = pricka / 2"
equation "d210 = pricka"
equation "d211 = mriz_y"
equation "d212 = pricka / 2"
equation "d213 = pricka / 2"
equation "d214 = -okraj"
equation "d216 = -kamera_sirka - okraj"

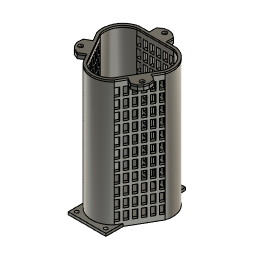
design "baterie_drzak"
Autodesk Fusion 360 part; units mm, degrees
sketch "Sketch2" plane through (0, 0, 0) normal (0, 0, 1) x (1, 0, 0)
  line L0 (-10.75, 0) -> (10.75, 0)
  line L1 (7.7886, -32.1098) -> (18.5386, -13.4902)
  line L2 (0, -15.2) -> (13.1636, -22.8) construction
  line L3 (0, 0) -> (0, -15.2) construction
  line L4 (-18.5386, -13.4902) -> (-7.7886, -32.1098)
  line L5 (-13.1636, -22.8) -> (0, -15.2) construction
  line L6 (0, -15.2) -> (-57.817, 18.1806) construction
  line L7 (0, -15.2) -> (57.1264, 17.782) construction
  line L8 (0, -15.2) -> (0, -80) construction
  circle A0 centre (-8.5459, -10.266) radius 10.5
  circle A1 centre (0, -25.0679) radius 10.5
  circle A2 centre (8.5459, -10.266) radius 10.5
  point P0 (0, -15.2)
  point P1 (13.1636, -22.8)
  point P2 (-13.1636, -22.8)
  dimension "d9" = 21.5
  dimension "d10" = 15.2
  dimension "d11" = 60
  dimension "d12" = 21.5
  dimension "d13" = 15.2
  dimension "d14" = 60
  dimension "d15" = 21.5
  dimension "d16" = 15.2
  dimension "d18" = 21
  dimension "d19" = 10.5
  dimension "d21" = 360
  constraint horizontal L0
  constraint midpoint L3.start L0
  constraint midpoint L1 P1
  constraint coincident P0 L2.start
  constraint coincident P1 L2.end
  constraint coincident L3.start origin
  constraint perpendicular L0 L3
  constraint perpendicular L1 L2
  constraint midpoint L4 P2
  constraint coincident P2 L5.start
  constraint perpendicular L4 L5
  constraint parallel L2 L6
  constraint parallel L5 L7
  constraint vertical L8
  constraint coincident L6 A0.centre
  measures "d9" distance of L0.start L0.end
  measures "d10" distance of L0 P0
  measures "d11" angle of L0 L1
  measures "d12" distance of L1.start L1.end
  measures "d13" distance of P0 P1
  measures "d14" angle of L0 L4
  measures "d15" distance of L4.start L4.end
  measures "d16" distance of P2 P0
  measures "d18" diameter of A0
  measures "d19" distance of L4.start A0.centre
extrude "Extrude2" add sketch "Sketch2" along normal blind 72.5 contours L0 L4 A0 A1 A2 | L0 A0 A2 | L0 L1 A0 A1 A2 | A0 A1 A2 | L4 A0 A1 | A0 A1 A2 | A0 A1 A2 | L1 L4 A0 A1 A2 | A0 A1 A2 | L1 A1 A2 makes body 1
sketch "Sketch3" plane through (0, 0, 72.5) normal (0, 0, 1) x (-1, 0, 0)
  arc A0 (10.75, 0) -> (18.5386, 13.4902) centre (8.5459, 10.266) ccw
  line L0 (18.5386, 13.4902) -> (7.7886, 32.1098)
  arc A1 (7.7886, 32.1098) -> (-7.7886, 32.1098) centre (0, 25.0679) ccw
  line L1 (-7.7886, 32.1098) -> (-18.5386, 13.4902)
  arc A2 (-18.5386, 13.4902) -> (-10.75, 0) centre (-8.5459, 10.266) ccw
  line L2 (-10.75, 0) -> (10.75, 0)
  line L3 (-10.7606, -0.1) -> (10.7606, -0.1)
  arc A3 (10.7606, -0.1) -> (18.6305, 13.5311) centre (8.5459, 10.266) ccw
  line L4 (18.6305, 13.5311) -> (7.8699, 32.1689)
  arc A4 (7.8699, 32.1689) -> (-7.8699, 32.1689) centre (0, 25.0679) ccw
  line L5 (-7.8699, 32.1689) -> (-18.6305, 13.5311)
  arc A5 (-18.6305, 13.5311) -> (-10.7606, -0.1) centre (-8.5459, 10.266) ccw
  dimension "d25" = 0.1
extrude "Extrude3" add sketch "Sketch3" against normal blind 72.5 contours A0 L0 A1 L1 A2 L2 | L3 A3 L4 A4 L5 A5 bodies 1
shell "Shell1" thickness 1.5 outward yes removed faces 1 at (0, -15.2, 72.5) on bodies 1